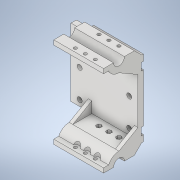
# Autodesk Inventor part: ZY_rod_mount
Saved by Autodesk Inventor 2020 (Build 240168000, 168)
## iProperties
Created: 2020-08-11
Part Number: ZY_rod_mount
Material: Tworzywo sztuczne ABS
Document SubType Name: Modeling
Designer: invin
Density: 1.06 g/cm^3
Appearance: Gładki — biały
Mass: 76.1571 g
Surface Area: 282.417 cm^2
Volume: 71.8463 cm^3
Author: invin
Autodesk Inventor part; units mm, degrees
sketch "Szkic1" plane through (0, 0, 0) normal (0, 0, 1) x (1, 0, 0)
  line L0 (0, 0) -> (74, 0)
  line L1 (74, 0) -> (74, 74)
  line L2 (74, 74) -> (0, 74)
  line L3 (0, 74) -> (0, 0)
  dimension "d0" = 74
  dimension "d1" = 74
  constraints: 8 end point, 2 parallel, 1 horizontal, 1 perpendicular
  measures "d0" distance of L1.end L2.end
  measures "d1" distance of L2.end L0.start
extrude "Wyciągnięcie proste1" add sketch "Szkic1" along normal blind 25
sketch "Szkic2" plane through (0, 0, 25) normal (0, 0, 1) x (1, 0, 0)
  line L0 (-55.7627, 31) -> (170, 31)
  line L1 (170, 31) -> (170, 11)
  line L2 (170, 11) -> (-55.7627, 11)
  line L3 (-55.7627, 11) -> (-55.7627, 31)
  line L4 (-31.3559, 63) -> (141.1864, 63)
  line L5 (141.1864, 63) -> (141.1864, 43)
  line L6 (141.1864, 43) -> (-31.3559, 43)
  line L7 (-31.3559, 43) -> (-31.3559, 63)
  line L8 (0, 0) -> (74, 0) projected
  line L9 (74, 74) -> (0, 74) projected
  dimension "d4" = 20
  dimension "d6" = 20
  dimension "d7" = 11
  dimension "d8" = 11
  constraints: 16 end point, 4 parallel, 2 horizontal, 2 perpendicular
  measures "d4" distance between parallel lines of L4 L6
  measures "d6" distance between parallel lines of L2 L0
  measures "d7" distance between parallel lines of L8 L2
  measures "d8" distance between parallel lines of L9 L4
extrude "Wyciągnięcie proste2" cut sketch "Szkic2" against normal blind 19.8
sketch "Szkic3" plane through (0, 0, 25) normal (0, 0, 1) x (1, 0, 0)
  line L0 (0, 9.95) -> (74, 9.95)
  line L1 (74, 9.95) -> (74, 2.05)
  line L2 (74, 2.05) -> (0, 2.05)
  line L3 (0, 2.05) -> (0, 9.95)
  line L4 (0, 71.95) -> (74, 71.95)
  line L5 (74, 71.95) -> (74, 64.05)
  line L6 (74, 64.05) -> (0, 64.05)
  line L7 (0, 64.05) -> (0, 71.95)
  line L8 (74, 74) -> (0, 74) projected
  line L9 (0, 74) -> (0, 63) projected
  line L10 (74, 63) -> (74, 74) projected
  line L11 (0, 0) -> (74, 0) projected
  line L12 (0, 11) -> (0, 0) projected
  line L13 (74, 0) -> (74, 11) projected
  dimension "d11" = 2.05
  dimension "d12" = 7.9
  dimension "d13" = 0
  dimension "d14" = 0
  dimension "d15" = 2.05
  dimension "d16" = 7.9
  dimension "d17" = 0
  dimension "d18" = 0
  constraints: 16 end point, 4 parallel, 2 horizontal, 2 perpendicular
  measures "d11" distance between parallel lines of L8 L4
  measures "d12" distance between parallel lines of L4 L6
  measures "d13" distance between parallel lines of L9 L7
  measures "d14" distance between parallel lines of L10 L5
  measures "d15" distance between parallel lines of L11 L2
  measures "d16" distance between parallel lines of L2 L0
  measures "d17" distance between parallel lines of L12 L3
  measures "d18" distance between parallel lines of L13 L1
extrude "Wyciągnięcie proste3" add sketch "Szkic3" along normal blind 1.9 contours L0 L1 L2 L3 | L4 L5 L6 L7
sketch "Szkic4" plane through (0, 0, 0) normal (-1, 0, 0) x (0, 0, 1)
  line L0 (0, 74) -> (25, 74) projected
  line L1 (0, 74) -> (0, 0) projected
  line L2 (25, 74) -> (0, 74)
  line L3 (0, 74) -> (0, 0)
  line L4 (0, 0) -> (25, 0)
  line L5 (25, 0) -> (25, 74)
  constraints: 8 end point, 2 parallel, 1 horizontal, 1 perpendicular
extrude "Wyciągnięcie proste4" add sketch "Szkic4" against normal blind 4
ref_plane "Płaszczyzna konstrukcyjna1" through (37, 0, 0) normal (1, 0, 0) x (0, 0, -1)
sketch "Szkic5" plane through (0, 0, 26.9) normal (0, 0, 1) x (1, 0, 0)
  circle A0 centre (9.61, 6) radius 2.75
  circle A1 centre (64.39, 6) radius 2.75
  line L0 (0, 0) -> (74, 0) projected
  line L1 (37, 88.8) -> (37, -14.8) projected
  dimension "d23" = 5.5
  dimension "d24" = 5.5
  dimension "d25" = 6
  dimension "d26" = 6
  dimension "d27" = 54.78
  dimension "d29" = 27.39
  constraints: 2 centre point
  measures "d23" diameter of A0
  measures "d24" diameter of A1
  measures "d25" distance from line of L0 A1.centre
  measures "d26" distance from line of L0 A0.centre
  measures "d27" distance of A1.centre A0.centre
  measures "d29" distance from line of L1 A0.centre
extrude "Wyciągnięcie proste5" cut sketch "Szkic5" against normal blind 50
pattern_linear "Szyk prostokątny1" count 3 spacing 31 along (0, 1, 0) of "Wyciągnięcie proste5"
chamfer "Faza1" distance 2 angle 45 8 edges at (0, 37, 25) (0, 72.975, 25) (0, 1.025, 25) (74, 1.025, 25) (74, 10.475, 25) (74, 37, 25) (74, 63.525, 25) (74, 72.975, 25)
chamfer "Faza2" distance 3.8999 angle 45 2 edges at (0, 6, 26.9) (0, 68, 26.9)
chamfer "Faza3" distance 3.8999 angle 45 2 edges at (74, 6, 26.9) (74, 68, 26.9)
sketch "Szkic6" plane through (0, 0, 26.9) normal (0, 0, 1) x (1, 0, 0)
  line L0 (-37.7989, 82.8258) -> (109.7385, 82.8258)
  line L1 (109.7385, 82.8258) -> (109.7385, -18.0074)
  line L2 (109.7385, -18.0074) -> (-37.7989, -18.0074)
  line L3 (-37.7989, -18.0074) -> (-37.7989, 82.8258)
  point P0 (0, 0)
  constraints: 8 end point, 2 parallel, 1 horizontal, 1 perpendicular
extrude "Wyciągnięcie proste6" cut sketch "Szkic6" against normal blind 22.9
sketch "Szkic7" plane through (74, 0, 0) normal (1, 0, 0) x (0, 0, -1)
  circle A0 centre (-25, 87) radius 6
  circle A1 centre (-25, -13) radius 6
  line L0 (0, 74) -> (-4, 74) projected
  line L1 (0, 0) -> (-4, 0) projected
  line L2 (0, 0) -> (0, 74) projected
  circle A2 centre (-25, 87) radius 12.5
  circle A3 centre (-25, -13) radius 12.5
  line L3 (-31, 87) -> (-37.5, 87)
  line L4 (-19, 87) -> (-12.5, 87)
  line L5 (-12.5, -13) -> (-19, -13)
  line L6 (-31, -13) -> (-37.5, -13)
  dimension "d46" = 12
  dimension "d47" = 12
  dimension "d48" = 100
  dimension "d49" = 13
  dimension "d50" = 13
  dimension "d51" = 25
  dimension "d52" = 25
  dimension "d53" = 25
  constraints: 8 end point, 8 point on circle, 4 centre point, 4 point on line, 2 coincident, 1 horizontal, 1 parallel
  measures "d46" diameter of A0
  measures "d47" diameter of A1
  measures "d48" distance of A0.centre A1.centre
  measures "d49" distance from line of L0 A0.centre
  measures "d50" distance from line of L1 A1.centre
  measures "d51" distance from line of A0.centre L2
  measures "d52" diameter of A2
  measures "d53" diameter of A3
extrude "Wyciągnięcie proste7" add sketch "Szkic7" against normal blind 55 contours L4 A2 L3 A0 | A1 L6 A3 L5 picked at (-14.7877, 86.0029) picked at (-35.1541, -11.5242)
sketch "Szkic8" plane through (74, 0, 0) normal (1, 0, 0) x (0, 0, -1)
  line L0 (0, 0) -> (-4, 0) projected
  line L1 (-4, 0) -> (0, 0)
  line L2 (0, 0) -> (0, -0.5)
  line L3 (0, -0.5) -> (-4, -0.5)
  line L4 (-4, -0.5) -> (-4, 0)
  line L5 (0, 0) -> (0, 74) projected
  line L6 (-4, 74) -> (0, 74)
  line L7 (0, 74) -> (0, 74.5)
  line L8 (0, 74.5) -> (-4, 74.5)
  line L9 (-4, 74.5) -> (-4, 74)
  dimension "d56" = 0
  dimension "d57" = 0.5
  dimension "d58" = 0.5
  constraints: 16 end point, 4 parallel, 2 horizontal, 2 perpendicular
  measures "d56" distance between parallel lines of L5 L2
  measures "d57" distance between parallel lines of L0 L3
  measures "d58" distance of L6.end L7.end
extrude "Wyciągnięcie proste8" add sketch "Szkic8" against normal blind 74
sketch "Szkic9" plane through (74, -0.5, 4) normal (1, 0, 0) x (0, 0, -1)
  line L0 (4, 0) -> (0, 0) projected
  line L1 (4, 0) -> (-21, 0)
  arc A0 (-8.5, -12.5) -> (-33.5, -12.5) centre (-21, -12.5) ccw projected
  line L2 (-21, 0) -> (-8.5, -12.5)
  line L3 (-8.5, -12.5) -> (4, -12.5)
  line L4 (4, -12.5) -> (4, 0)
  point P0 (4, 0.5)
  constraints: 8 end point, 1 parallel, 1 perpendicular, 1 point on circle, 1 tangent
extrude "Wyciągnięcie proste9" add sketch "Szkic9" against normal blind 55 contours L4 L3 A0 L1 L0
sketch "Szkic10" plane through (74, -13, 25) normal (1, 0, 0) x (0, 0, -1)
  line L0 (25, 87.5) -> (25, 0) projected
  line L1 (25, 87.5) -> (0, 87.5)
  arc A0 (-12.5, 100) -> (12.5, 100) centre (0, 100) ccw projected
  line L2 (6, 100) -> (12.5, 100) projected
  line L3 (0, 87.5) -> (12.5, 100)
  line L4 (12.5, 100) -> (25, 100)
  line L5 (25, 87.5) -> (21, 87.5) projected
  line L6 (25, 87.5) -> (25, 100)
  point P0 (25, 13)
  constraints: 8 end point, 1 parallel, 1 perpendicular, 1 point on circle, 1 tangent
extrude "Wyciągnięcie proste10" add sketch "Szkic10" against normal blind 55
sketch "Szkic12" plane through (74, -13, 0) normal (0, -1, 0) x (1, 0, 0)
  circle A0 centre (-13.1, 12) radius 1.75
  line L0 (0, 19) -> (0, 0) projected
  line L1 (0, 25) -> (-55, 25) projected
  point P0 (-74, 0)
  dimension "d65" = 3.5
  dimension "d66" = 13.1
  dimension "d67" = 13
  constraints: 1 centre point
  measures "d65" diameter of A0
  measures "d66" distance from line of L0 A0.centre
  measures "d67" distance from line of L1 A0.centre
extrude "Wyciągnięcie proste11" cut sketch "Szkic12" against normal blind 5000
pattern_linear "Szyk prostokątny2" count 3 spacing 11 along (-1, 0, 0) of "Wyciągnięcie proste11"
sketch "Szkic13" plane through (74, -13, 25) normal (1, 0, 0) x (0, 0, -1)
  arc A0 (6, 0) -> (-6, 0) centre (0, 0) ccw projected
  line L0 (-6, 0) -> (-17, 0)
  line L1 (-17, 0) -> (-17, 5)
  line L2 (-17, 5) -> (-6, 5)
  line L3 (-6, 5) -> (-6, 0)
  line L4 (-6, 100) -> (-12.5, 100) projected
  line L5 (-6, 100) -> (-17, 100)
  line L6 (-17, 100) -> (-17, 95)
  line L7 (-17, 95) -> (-6, 95)
  line L8 (-6, 95) -> (-6, 100)
  point P0 (25, 13)
  dimension "d73" = 11
  dimension "d74" = 11
  dimension "d75" = 5
  dimension "d76" = 5
  constraints: 16 end point, 4 parallel, 2 horizontal, 2 perpendicular
  measures "d73" distance between parallel lines of L3 L1
  measures "d74" distance of L7.end L6.end
  measures "d75" distance between parallel lines of L5 L7
  measures "d76" distance of L0.end L1.end
extrude "Wyciągnięcie proste12" add sketch "Szkic13" against normal blind 55
ref_plane "Płaszczyzna konstrukcyjna2" through (0, 0, 25) normal (0, 0, -1) x (-1, 0, 0)
mirror "Odbij1" about plane through (0, 0, 25) normal (0, 0, -1) of "Wyciągnięcie proste11", "Szyk prostokątny2"
chamfer "Faza4" distance 8 angle 45 2 edges at (46.5, -13, 0) (46.5, 87, 0)
sketch "Szkic15" plane through (74, 74.5, 4) normal (0, -1, 0) x (1, 0, 0)
  circle A0 centre (-13.1, 8) radius 2.8
  circle A1 centre (-13.1, 8) radius 1.75 projected
  line L0 (-13.1, 5.2) -> (-15.5249, 6.6)
  line L1 (-15.5249, 6.6) -> (-15.5249, 9.4)
  line L2 (-15.5249, 9.4) -> (-13.1, 10.8)
  line L3 (-13.1, 10.8) -> (-10.6751, 9.4)
  line L4 (-10.6751, 9.4) -> (-10.6751, 6.6)
  line L5 (-10.6751, 6.6) -> (-13.1, 5.2)
  line L6 (0, 0) -> (-55, 0) projected
  point P0 (-74, -4)
  dimension "d83" = 5.6
  dimension "d84" = 90
  constraints: 12 end point, 1 coincident, 1 vertical alignment, 16 other
  measures "d84" angle of L6 L1
extrude "Wyciągnięcie proste13" cut sketch "Szkic15" against normal blind 8 contours L4 L5 L0 L1 L2 L3
pattern_linear "Szyk prostokątny3" count 3 spacing 11 along (-1, 0, 0) of "Wyciągnięcie proste13"
sketch "Szkic16" plane through (74, 82, 36.4564) normal (0, -1, 0) x (1, 0, 0)
  circle A0 centre (-35.1, 1.5436) radius 4
  arc A1 (-34.2754, 0) -> (-35.9246, 0) centre (-35.1, 1.5436) ccw projected
  point P0 (-74, -36.4564)
  dimension "d90" = 8
  constraints: 1 centre point, 1 concentric
  measures "d90" diameter of A0
extrude "Wyciągnięcie proste14" cut sketch "Szkic16" along normal blind 8
pattern_linear "Szyk prostokątny4" count 3 spacing 11 along (1, 0, 0) of "Wyciągnięcie proste14"
sketch "Szkic17" plane through (74, -8, 42) normal (0, 1, 0) x (1, 0, 0)
  circle A0 centre (-35.1, 4) radius 4
  arc A1 (-35.9246, 5.5436) -> (-34.2754, 5.5436) centre (-35.1, 4) ccw projected
  point P0 (-74, 42)
  dimension "d96" = 8
  constraints: 1 centre point, 1 concentric
  measures "d96" diameter of A0
extrude "Wyciągnięcie proste15" cut sketch "Szkic17" along normal blind 8
pattern_linear "Szyk prostokątny5" count 3 spacing 11 along (1, 0, 0) of "Wyciągnięcie proste15"
sketch "Szkic18" plane through (74, 87, 25) normal (1, 0, 0) x (0, 0, -1)
  line L0 (21, -87.5) -> (0, -87.5) projected
  line L1 (0, -87.5) -> (21, -75.3756)
  line L2 (21, -12.5) -> (21, -87.5) projected
  line L3 (21, -75.3756) -> (21, -87.5)
  line L4 (21, -87.5) -> (0, -87.5)
  line L5 (0, -12.5) -> (21, -12.5) projected
  line L6 (0, -12.5) -> (21, -12.5)
  line L7 (21, -12.5) -> (21, -24.6244)
  line L8 (0, -12.5) -> (21, -24.6244)
  point P0 (25, -87)
  dimension "d102" = 30
  dimension "d103" = 30
  constraints: 12 end point, 2 point on line, 1 horizontal, 1 perpendicular, 1 vertical
  measures "d102" angle of L5 L8
  measures "d103" angle of L0 L1
extrude "Wyciągnięcie proste16" add sketch "Szkic18" against normal blind 4
ref_plane "Płaszczyzna konstrukcyjna4" through (19, 37, 31) normal (0, 1, 0) x (1, 0, 0)
mirror "Odbij3" about plane through (19, 37, 31) normal (0, 1, 0) of "Wyciągnięcie proste13", "Szyk prostokątny3"
pattern_linear "Szyk prostokątny6" count 2 spacing 51 along (-1, 0, 0) of "Wyciągnięcie proste16"
sketch "Szkic20" plane through (74, 82, 42) normal (1, 0, 0) x (0, 0, -1)
  line L0 (48.2715, -80.05) -> (39.5, -80.05)
  line L1 (39.5, -80.05) -> (39.5, -71.95)
  line L2 (39.5, -71.95) -> (48.2715, -71.95)
  line L3 (48.2715, -71.95) -> (48.2715, -80.05)
  line L4 (51.3094, -18.05) -> (39.5, -18.05)
  line L5 (39.5, -18.05) -> (39.5, -9.95)
  line L6 (39.5, -9.95) -> (51.3094, -9.95)
  line L7 (51.3094, -9.95) -> (51.3094, -18.05)
  line L8 (42, -3) -> (42, -87) projected
  line L9 (57.0791, -76) -> (29.5355, -76)
  line L10 (-11.4158, -45) -> (68.4949, -45) projected
  point P0 (42, -82)
  dimension "d117" = 2.5
  dimension "d118" = 2.5
  dimension "d119" = 62
  dimension "d120" = 8.7715
  dimension "d121" = 8.1
  dimension "d122" = 8.1
  dimension "d123" = 4.05
  dimension "d124" = 31
  constraints: 18 end point, 4 parallel, 3 horizontal, 2 perpendicular
  measures "d117" distance between parallel lines of L1 L8
  measures "d118" distance between parallel lines of L5 L8
  measures "d119" distance between parallel lines of L4 L0
  measures "d120" distance of L0.start L0.end
  measures "d121" distance between parallel lines of L2 L0
  measures "d122" distance between parallel lines of L6 L4
  measures "d123" distance between parallel lines of L2 L9
  measures "d124" distance between parallel lines of L10 L9
extrude "Wyciągnięcie proste18" cut sketch "Szkic20" against normal blind 500
sketch "Szkic21" plane through (74, 82, 42) normal (1, 0, 0) x (0, 0, -1)
  line L0 (42, -80.05) -> (42, -87) projected
  line L1 (42, -87) -> (44, -87)
  line L2 (44, -87) -> (44, -3)
  line L3 (44, -3) -> (42, -3)
  line L4 (42, -3) -> (42, -87)
  line L5 (39.5, -18.05) -> (42, -18.05) projected
  line L6 (42, -7.5) -> (42, -9.95) projected
  line L7 (39.5, -18.05) -> (42, -18.05)
  line L8 (42, -18.05) -> (42, -9.95)
  line L9 (42, -9.95) -> (39.5, -9.95)
  line L10 (39.5, -9.95) -> (39.5, -18.05)
  line L11 (42, -80.05) -> (39.5, -80.05) projected
  line L12 (39.5, -71.95) -> (42, -71.95) projected
  line L13 (39.5, -80.05) -> (42, -80.05)
  line L14 (42, -80.05) -> (42, -71.95)
  line L15 (42, -71.95) -> (39.5, -71.95)
  line L16 (39.5, -71.95) -> (39.5, -80.05)
  point P0 (42, -82)
  dimension "d127" = 84
  dimension "d128" = 2
  constraints: 24 end point, 6 parallel, 3 horizontal, 3 perpendicular
  measures "d127" distance between parallel lines of L1 L3
  measures "d128" distance between parallel lines of L4 L2
extrude "Wyciągnięcie proste19" add sketch "Szkic21" against normal blind 74
sketch "Szkic22" plane through (0, 79, 0) normal (0, 0, 1) x (1, 0, 0)
  line L0 (19, -16.6244) -> (19, -4.5) projected
  line L1 (19, -4.5) -> (-9.5464, -4.5)
  line L2 (-9.5464, -4.5) -> (-9.5464, 5.3732)
  line L3 (-9.5464, 5.3732) -> (19, 5.3732)
  line L4 (19, 5.3732) -> (19, -4.5)
  line L5 (19, -79.5) -> (0, -79.5) projected
  line L6 (19, -79.5) -> (-15.8101, -79.5)
  line L7 (-15.8101, -79.5) -> (-15.8101, -92.9885)
  line L8 (-15.8101, -92.9885) -> (19, -92.9885)
  line L9 (19, -92.9885) -> (19, -79.5)
  point P0 (0, -79)
  constraints: 16 end point, 4 parallel, 2 horizontal, 2 perpendicular
extrude "Wyciągnięcie proste20" cut sketch "Szkic22" against normal blind 74
sketch "Szkic23" plane through (0, 0, 4) normal (0, 0, 1) x (1, 0, 0)
  circle A0 centre (9.61, 6) radius 2.75
  circle A1 centre (9.61, 37) radius 2.75 projected
  circle A2 centre (9.61, 37) radius 2.75
  circle A3 centre (64.39, 6) radius 2.75
  circle A4 centre (64.39, 37) radius 2.75
  circle A5 centre (64.39, 68) radius 2.75
  circle A6 centre (9.61, 68) radius 2.75
  circle A7 centre (9.61, 68) radius 2.75 projected
  circle A8 centre (9.61, 6) radius 2.75 projected
  circle A9 centre (64.39, 6) radius 2.75 projected
  circle A10 centre (64.39, 37) radius 2.75 projected
  circle A11 centre (64.39, 68) radius 2.75 projected
  point P0 (0, 0)
  dimension "d133" = 5.5
  dimension "d134" = 5.5
  dimension "d135" = 5.5
  dimension "d136" = 5.5
  dimension "d137" = 5.5
  dimension "d138" = 5.5
  constraints: 6 centre point, 5 concentric, 1 coincident
  measures "d133" diameter of A0
  measures "d134" diameter of A2
  measures "d135" diameter of A3
  measures "d136" diameter of A4
  measures "d137" diameter of A5
  measures "d138" diameter of A6
extrude "Wyciągnięcie proste21" cut sketch "Szkic23" against normal blind 74
sketch "Szkic24" plane through (74, 82, 42) normal (1, 0, 0) x (0, 0, -1)
  line L0 (45.4172, -80.05) -> (41.5, -80.05)
  line L1 (41.5, -80.05) -> (41.5, -71.95)
  line L2 (41.5, -71.95) -> (45.4172, -71.95)
  line L3 (45.4172, -71.95) -> (45.4172, -80.05)
  line L4 (46.4297, -18.05) -> (41.5, -18.05)
  line L5 (41.5, -18.05) -> (41.5, -9.95)
  line L6 (41.5, -9.95) -> (46.4297, -9.95)
  line L7 (46.4297, -9.95) -> (46.4297, -18.05)
  line L8 (49.5433, -76) -> (34.2517, -76)
  line L9 (-9.9087, -45) -> (59.452, -45) projected
  line L10 (44, -87) -> (44, -3) projected
  point P0 (42, -82)
  dimension "d141" = 8.1
  dimension "d142" = 8.1
  dimension "d143" = 62
  dimension "d144" = 4.05
  dimension "d145" = 31
  dimension "d146" = 2.5
  constraints: 18 end point, 4 parallel, 3 horizontal, 2 perpendicular, 1 point on line
  measures "d141" distance of L0.end L1.end
  measures "d142" distance of L4.end L5.end
  measures "d143" distance between parallel lines of L6 L2
  measures "d144" distance between parallel lines of L2 L8
  measures "d145" distance between parallel lines of L9 L8
  measures "d146" distance between parallel lines of L10 L1
extrude "Wyciągnięcie proste22" cut sketch "Szkic24" against normal blind 74
